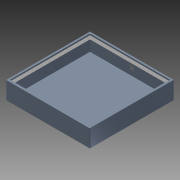
# Autodesk Inventor part: Propane Burner
Saved by Autodesk Inventor 2013 SP2 (Build 170200200, 200)
## iProperties
Created: 2014-05-29
Part Number: Propane Burner
Material: Steel
Document SubType Name: Modeling
Designer: rmclane
Density: 7.85 g/cm^3
Mass: 5958.17 g
Surface Area: 9072.97 cm^2
Volume: 759.002 cm^3
Author: rmclane
Autodesk Inventor part; units mm, degrees
ref_plane "YZ Plane" through (0, 0, 0) normal (1, 0, 0) x (0, 1, 0)
ref_plane "XZ Plane" through (0, 0, 0) normal (0, 1, 0) x (-1, 0, 0)
sketch "Sketch1" plane through (0, 0, 0) normal (0, 1, 0) x (-1, 0, 0)
  line L0 (-462.2267, 0) -> (462.2267, 0) projected
  line L1 (0, -462.2267) -> (0, 462.2267) projected
  line L2 (-330.1619, 330.1619) -> (330.1619, 330.1619)
  line L3 (330.1619, 330.1619) -> (330.1619, -330.1619)
  line L4 (330.1619, -330.1619) -> (-330.1619, -330.1619)
  line L5 (-330.1619, -330.1619) -> (-330.1619, 330.1619)
  line L6 (462.2267, 0) -> (-462.2267, 0) projected
  line L7 (0, -462.2267) -> (0, 462.2267) projected
  line L8 (314.2869, -314.2869) -> (-314.2869, -314.2869)
  line L9 (-314.2869, -314.2869) -> (-314.2869, 314.2869)
  line L10 (-314.2869, 314.2869) -> (314.2869, 314.2869)
  line L11 (314.2869, 314.2869) -> (314.2869, -314.2869)
  point P0 (0, 0)
  dimension "d0" = 660.3238
  dimension "d2" = 660.3238
  dimension "d123" = 15.875
  dimension "d124" = 15.875
  constraints: 16 end point, 4 parallel, 2 horizontal, 2 perpendicular, 4 other
  measures "d0" distance between parallel lines of L3 L5
  measures "d2" distance between parallel lines of L2 L4
  measures "d123" distance between parallel lines of L4 L8
  measures "d124" distance between parallel lines of L5 L9
extrude "Extrusion1" add sketch "Sketch1" against normal blind 1.5875 contours L5 L2 L1 L10 L9 L0 | L0 L9 L8 L1 L4 L5 | L1 L8 L11 L0 L3 L4 | L2 L3 L0 L11 L10 L1
sketch "Sketch2" plane through (0, -1.5875, 0) normal (0, -1, 0) x (1, 0, 0)
  line L0 (330.1619, 330.1619) -> (-330.1619, 330.1619) projected
  line L1 (-330.1619, 330.1619) -> (-330.1619, -330.1619) projected
  line L2 (-330.1619, -330.1619) -> (330.1619, -330.1619) projected
  line L3 (330.1619, -330.1619) -> (330.1619, 330.1619) projected
  line L4 (-314.2869, -314.2869) -> (-314.2869, 314.2869) projected
  line L5 (-314.2869, 314.2869) -> (314.2869, 314.2869) projected
  line L6 (314.2869, 314.2869) -> (314.2869, -314.2869) projected
  line L7 (314.2869, -314.2869) -> (-314.2869, -314.2869) projected
  line L8 (330.1619, 330.1619) -> (-330.1619, 330.1619) projected
  line L9 (-330.1619, 330.1619) -> (-330.1619, -330.1619) projected
  line L10 (-330.1619, -330.1619) -> (330.1619, -330.1619) projected
  line L11 (330.1619, -330.1619) -> (330.1619, 330.1619) projected
  line L12 (0, -462.2267) -> (0, 462.2267) projected
  line L13 (-462.2267, 0) -> (462.2267, 0) projected
  line L14 (-328.5744, 328.5744) -> (328.5744, 328.5744)
  line L15 (328.5744, 328.5744) -> (328.5744, -328.5744)
  line L16 (328.5744, -328.5744) -> (-328.5744, -328.5744)
  line L17 (-328.5744, -328.5744) -> (-328.5744, 328.5744)
  point P0 (0, 0)
  dimension "d7" = 1.5875
  dimension "d8" = 1.5875
  constraints: 8 end point, 2 parallel, 1 horizontal, 1 perpendicular, 2 other
  measures "d7" distance between parallel lines of L0 L14
  measures "d8" distance between parallel lines of L1 L17
extrude "Extrusion2" add sketch "Sketch2" along normal blind 136.525 contours L3 L13 L15 L14 L12 L0 | L12 L14 L17 L13 L1 L0 | L3 L2 L12 L16 L15 L13 | L13 L17 L16 L12 L2 L1
sketch "Sketch3" plane through (0, -138.1125, 0) normal (0, -1, 0) x (1, 0, 0)
  line L0 (-462.2267, 0) -> (462.2267, 0) projected
  line L1 (0, -462.2267) -> (0, 462.2267) projected
  line L2 (-330.1619, 330.1619) -> (330.1619, 330.1619)
  line L3 (330.1619, 330.1619) -> (330.1619, -330.1619)
  line L4 (330.1619, -330.1619) -> (-330.1619, -330.1619)
  line L5 (-330.1619, -330.1619) -> (-330.1619, 330.1619)
  point P0 (0, 0)
  constraints: 8 end point, 2 parallel, 1 horizontal, 1 perpendicular
extrude "Extrusion3" add sketch "Sketch3" along normal blind 1.5875
ref_plane "Work Plane1" through (0, -25.4, 0) normal (0, 1, 0) x (1, 0, 0)
sketch "Sketch4" plane through (0, -25.4, 0) normal (0, 1, 0) x (1, 0, 0)
  line L0 (328.5744, -328.5744) -> (328.5744, 328.5744) projected
  line L1 (328.5744, 328.5744) -> (-328.5744, 328.5744) projected
  line L2 (-328.5744, 328.5744) -> (-328.5744, -328.5744) projected
  line L3 (-328.5744, -328.5744) -> (328.5744, -328.5744) projected
  line L4 (-330.1619, -330.1619) -> (-330.1619, 330.1619) projected
  line L5 (-330.1619, 330.1619) -> (330.1619, 330.1619) projected
  line L6 (330.1619, 330.1619) -> (330.1619, -330.1619) projected
  line L7 (330.1619, -330.1619) -> (-330.1619, -330.1619) projected
  line L8 (-299.9994, 299.9994) -> (299.9994, 299.9994)
  line L9 (299.9994, 299.9994) -> (299.9994, -299.9994)
  line L10 (299.9994, -299.9994) -> (-299.9994, -299.9994)
  line L11 (-299.9994, -299.9994) -> (-299.9994, 299.9994)
  line L12 (462.2267, 0) -> (-462.2267, 0) projected
  line L13 (0, 462.2267) -> (0, -462.2267) projected
  point P0 (0, 0)
  dimension "d121" = 30.1625
  dimension "d122" = 30.1625
  constraints: 8 end point, 2 parallel, 1 horizontal, 1 perpendicular, 2 other
  measures "d121" distance between parallel lines of L8 L5
  measures "d122" distance between parallel lines of L4 L11
extrude "Extrusion4" add sketch "Sketch4" against normal blind 1.5875 contours L3 L13 L10 L9 L12 L0 | L12 L9 L8 L13 L1 L0 | L3 L2 L12 L11 L10 L13 | L13 L8 L11 L12 L2 L1
fillet "Fillet1" radius 3.175 12 edges at (0, 0, 330.1619) (0, -139.7, 330.1619) (330.1619, -69.85, 330.1619) (330.1619, -139.7, 0) (330.1619, 0, 0) (330.1619, -69.85, -330.1619) (0, 0, -330.1619) (-330.1619, 0, 0) (-330.1619, -69.85, 330.1619) (0, -139.7, -330.1619) (-330.1619, -69.85, -330.1619) (-330.1619, -139.7, 0)
sketch "Sketch5" plane through (330.1619, 0, -330.1619) normal (0, 0, -1) x (-1, 0, 0)
  line L0 (660.3238, -139.7) -> (0, -139.7) projected
  line L1 (330.1619, -167.64) -> (330.1619, 27.94) projected
  circle A0 centre (330.1619, -82.55) radius 16.7005
  line L2 (657.1488, 0) -> (3.175, 0) projected
  line L3 (3.175, -139.7) -> (657.1488, -139.7) projected
  point P0 (330.1619, 0)
  dimension "d74" = 57.15
  dimension "d75" = 33.401
  constraints: 1 centre point, 1 point on line
  measures "d74" distance from line of L0 A0.centre
  measures "d75" diameter of A0
extrude "Extrusion10" cut sketch "Sketch5" against normal up to surface (1.5875 mm away)
sketch "Sketch6" plane through (-328.5744, -138.1125, -328.5744) normal (0, 0, 1) x (1, 0, 0)
  circle A0 centre (298.4119, 42.8625) radius 15.875 projected
  circle A1 centre (298.4119, 42.8625) radius 15.875
  circle A2 centre (298.4119, 42.8625) radius 12.7
  point P0 (328.5744, 138.1125)
  dimension "d83" = 25.4
  constraints: 2 centre point, 2 coincident, 1 concentric
  measures "d83" diameter of A2
sketch "Sketch7" plane through (330.1619, -136.525, 326.9869) normal (1, 0, 0) x (0, 0, -1)
  line L0 (653.9738, 136.525) -> (0, 136.525) projected
  line L1 (326.9869, -31.115) -> (326.9869, 164.465) projected
  circle A0 centre (55.5752, 120.65) radius 3.175
  line L2 (-1.5875, 134.9375) -> (-1.5875, 111.125) projected
  line L3 (-3.175, 133.35) -> (-3.175, 0) projected
  circle A1 centre (598.3986, 120.65) radius 3.175
  point P0 (326.9869, 136.525)
  dimension "d91" = 6.35
  dimension "d95" = 58.7502
  dimension "d96" = 15.875
  constraints: 2 centre point, 1 symmetric about line, 1 other
  measures "d91" diameter of A0
  measures "d95" distance from line of L3 A0.centre
  measures "d96" distance from line of L0 A0.centre
body "Solid1"
